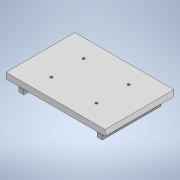
# Autodesk Inventor part: Soporte de matriz
Saved by Autodesk Inventor 2021 (Build 250183000, 183)
## iProperties
Created: 2021-06-06
Part Number: Soporte de matriz
Material: Generic
Document SubType Name: Modeling
Designer: Nelson
Density: 1 g/cm^3
Appearance: Default
Author: Nelson
Autodesk Inventor part; units mm, degrees
ref_plane "YZ Plane" through (0, 0, 0) normal (1, 0, 0) x (0, 1, 0)
ref_plane "XZ Plane" through (0, 0, 0) normal (0, 1, 0) x (-1, 0, 0)
ref_plane "XY Plane" through (0, 0, 0) normal (0, 0, 1) x (1, 0, 0)
sketch "Sketch1" plane through (0, 0, 0) normal (0, 1, 0) x (-1, 0, 0)
  line L0 (0, 0) -> (-506.2, 0)
  line L1 (-506.2, 0) -> (-506.2, -351.6)
  line L2 (-506.2, -351.6) -> (0, -351.6)
  line L3 (0, -351.6) -> (0, 0)
  dimension "d0" = 506.2
  dimension "d1" = 351.6
  constraints: 8 end point, 2 parallel, 1 horizontal, 1 perpendicular
  measures "d0" distance of L2.end L1.end
  measures "d1" distance of L1.end L0.end
extrude "Extrusion1" add sketch "Sketch1" against normal blind 30
sketch "Sketch2" plane through (0, -30, 0) normal (0, -1, 0) x (1, 0, 0)
  line L0 (466.2, -326.2) -> (440.8, -326.2)
  line L1 (440.8, -326.2) -> (440.8, -25.4)
  line L2 (440.8, -25.4) -> (466.2, -25.4)
  line L3 (466.2, -25.4) -> (466.2, -326.2)
  line L4 (65.4, -326.2) -> (40, -326.2)
  line L5 (40, -326.2) -> (40, -25.4)
  line L6 (40, -25.4) -> (65.4, -25.4)
  line L7 (65.4, -25.4) -> (65.4, -326.2)
  line L8 (506.2, 0) -> (0, 0) projected
  line L9 (0, -351.6) -> (506.2, -351.6) projected
  line L10 (0, 0) -> (0, -351.6) projected
  dimension "d4" = 25.4
  dimension "d5" = 25.4
  dimension "d6" = 25.4
  dimension "d7" = 25.4
  dimension "d9" = 25.4
  dimension "d10" = 25.4
  dimension "d11" = 40
  dimension "d12" = 375.4
  constraints: 16 end point, 4 parallel, 2 horizontal, 2 perpendicular, 2 point on line
  measures "d4" distance between parallel lines of L2 L8
  measures "d5" distance between parallel lines of L6 L8
  measures "d6" distance between parallel lines of L0 L9
  measures "d7" distance between parallel lines of L4 L9
  measures "d9" distance between parallel lines of L1 L3
  measures "d10" distance between parallel lines of L5 L7
  measures "d11" distance between parallel lines of L10 L5
  measures "d12" distance between parallel lines of L7 L1
extrude "Extrusion2" add sketch "Sketch2" along normal blind 50
sketch "Sketch4" plane through (0, 0, 0) normal (0, 1, 0) x (1, 0, 0)
  line L0 (0, 351.6) -> (0, 0) projected
  line L1 (506.2, 351.6) -> (0, 351.6) projected
  line L2 (506.2, 0) -> (506.2, 351.6) projected
  point P0 (138.1, 258.3)
  point P1 (368.1, 258.3)
  point P2 (138.1, 93.3)
  point P3 (368.1, 93.3)
  dimension "d22" = 230
  dimension "d23" = 230
  dimension "d24" = 165
  dimension "d25" = 165
  dimension "d26" = 138.1
  dimension "d27" = 138.1
  dimension "d28" = 93.3
  dimension "d36" = 93.3
  measures "d22" distance of point (368.1, 258.3) point (138.1, 258.3)
  measures "d23" distance of point (368.1, 93.3) point (138.1, 93.3)
  measures "d24" distance of point (138.1, 93.3) point (138.1, 258.3)
  measures "d25" distance of point (368.1, 93.3) point (368.1, 258.3)
  measures "d26" distance from line of point (138.1, 93.3) L0
  measures "d27" distance from line of point (138.1, 258.3) L0
  measures "d28" distance from line of point (138.1, 258.3) L1
  measures "d36" distance from line of point (368.1, 258.3) L1
hole "Hole1" at (138.1, 0, -258.3) at (368.1, 0, -258.3) at (138.1, 0, -93.3) at (368.1, 0, -93.3) direction (0, -1, 0) diameter 11.835 depth 12 tip angle 137 thread size "M14x2" class "6H" standard "ISO Metric profile"
equation "\"d6\" = d4"
equation "\"d10\" = d9"
equation "\"d23\" = d22"
equation "\"d25\" = d24"
equation "\"d27\" = d26"
equation "\"d36\" = d28"
body "Solid1"
